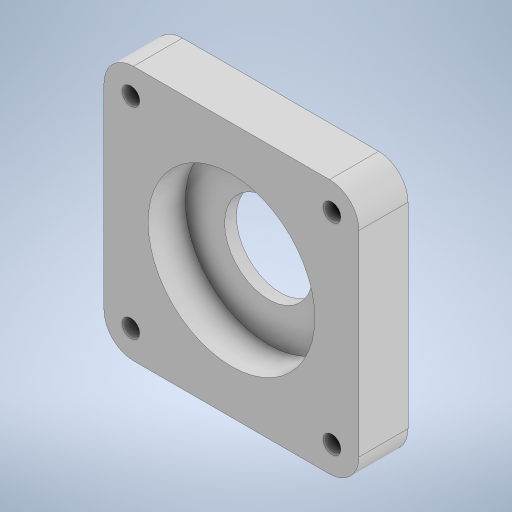
# Autodesk Inventor part: EndEffectorMotorAdapter
Saved by Autodesk Inventor 2024 (Build 280153000, 153)
## iProperties
Created: 2024-02-13
Part Number: EndEffectorMotorAdapter
Material: Generic
Document SubType Name: Modeling
Designer: yusuf
Density: 1 g/cm^3
Appearance: Default
Author: yusuf
Autodesk Inventor part; units mm, degrees
ref_plane "YZ Plane" through (0, 0, 0) normal (1, 0, 0) x (0, 1, 0)
ref_plane "XZ Plane" through (0, 0, 0) normal (0, 1, 0) x (-1, 0, 0)
ref_plane "XY Plane" through (0, 0, 0) normal (0, 0, 1) x (1, 0, 0)
sketch "Sketch6" plane through (0, 0, 0) normal (0, 0, 1) x (1, 0, 0)
  line L0 (0, 0) -> (130, 0)
  line L1 (130, 0) -> (130, 130)
  line L2 (130, 130) -> (0, 130)
  line L3 (0, 130) -> (0, 0)
  circle A0 centre (65, 65) radius 42.5
  dimension "d28" = 130
  dimension "d29" = 130
  dimension "d30" = 85
  dimension "d31" = 65
  dimension "d32" = 65
  constraints: 8 end point, 2 parallel, 1 centre point, 1 horizontal, 1 perpendicular
  measures "d28" distance of L1.end L2.end
  measures "d29" distance of L0.end L1.end
  measures "d30" diameter of A0
  measures "d31" distance from line of L3 A0.centre
  measures "d32" distance from line of L0 A0.centre
extrude "Extrusion6" add sketch "Sketch6" along normal blind 25
sketch "Sketch7" plane through (0, 0, 25) normal (0, 0, 1) x (1, 0, 0)
  circle A0 centre (116.265, 116.265) radius 4.5
  line L0 (130, 0) -> (130, 130) projected
  circle A1 centre (65, 65) radius 42.5 projected
  circle A2 centre (13.735, 116.265) radius 4.5
  circle A3 centre (13.735, 13.735) radius 4.5
  circle A4 centre (116.265, 13.735) radius 4.5
  point P0 (0, 0)
  dimension "d36" = 51.265
  dimension "d37" = 51.265
  dimension "d38" = 9
  dimension "d39" = 9
  dimension "d40" = 9
  dimension "d41" = 9
  dimension "d42" = 51.265
  dimension "d43" = 51.265
  dimension "d44" = 51.265
  dimension "d45" = 51.265
  dimension "d46" = 51.265
  dimension "d47" = 51.265
  constraints: 4 centre point
  measures "d36" horizontal distance of A0.centre A1.centre
  measures "d37" horizontal distance of A1.centre A0.centre
  measures "d38" diameter of A0
  measures "d39" diameter of A2
  measures "d40" diameter of A3
  measures "d41" diameter of A4
  measures "d42" horizontal distance of A2.centre A1.centre
  measures "d43" horizontal distance of A1.centre A2.centre
  measures "d44" horizontal distance of A1.centre A3.centre
  measures "d45" horizontal distance of A1.centre A3.centre
  measures "d46" horizontal distance of A1.centre A4.centre
  measures "d47" horizontal distance of A1.centre A4.centre
extrude "Extrusion7" cut sketch "Sketch7" against normal blind 25 contours A0 | A2 | A3 | A4
fillet "Fillet1" radius 15 4 edges at (0, 130, 12.5) (130, 130, 12.5) (130, 0, 12.5) (0, 0, 12.5)
sketch "Sketch9" plane through (0, 0, 0) normal (0, 0, -1) x (-1, 0, 0)
  circle A0 centre (-65, 65) radius 42.5 projected
  circle A1 centre (-65, 65) radius 42.5
  circle A2 centre (-65, 65) radius 22.5
  point P0 (0, 0)
  dimension "d54" = 85
  dimension "d55" = 45
  constraints: 2 centre point, 2 coincident
  measures "d54" diameter of A1
  measures "d55" diameter of A2
extrude "Extrusion9" add sketch "Sketch9" against normal blind 6
equation "\"d31\" = 0.5 * d28"
equation "\"d32\" = 0.5 * d29"
equation "\"d42\" = d36"
equation "\"d43\" = d36"
equation "\"d44\" = d36"
equation "\"d45\" = d36"
equation "\"d46\" = d36"
equation "\"d47\" = d36"
body "Solid2"
